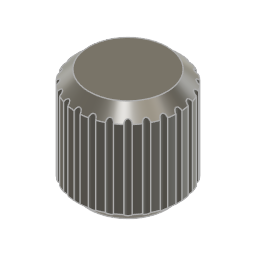
Shrimple20 Keypad Knob (Autodesk Fusion 360 design; units mm, degrees)
Autodesk Fusion 360 part; units mm, degrees
sketch "Sketch1" plane through (0, 0, 0) normal (0, 1, 0) x (1, 0, 0)
  circle A0 centre (0, 0) radius 8.5
  dimension "d1" = 17
  constraint coincident A0.centre origin
  measures "d1" diameter of A0
extrude "Extrude1" add sketch "Sketch1" along normal blind 17
ref_plane "WorkPlane1" through (0, 14, 0) normal (0, 1, 0) x (1, 0, 0)
sketch "Sketch2" plane through (0, 14, 0) normal (0, 1, 0) x (1, 0, 0)
  circle A0 centre (0, 0) radius 3.05
  line L0 (-0.5, 3.0087) -> (-0.5, -3.0087)
  line L1 (0.5, -3.0087) -> (0.5, 3.0087)
  line L2 (-0.5, 0) -> (0.5, 0) construction
  dimension "d5" = 6.1
  dimension "d6" = 1
  constraint coincident A0.centre origin
  constraint coincident A0 L0.start
  constraint coincident A0 L0.end
  constraint vertical L0
  constraint coincident A0 L1.start
  constraint coincident A0 L1.end
  constraint parallel L0 L1
  constraint midpoint L0 L2.start
  constraint midpoint L1 L2.end
  constraint midpoint A0.centre L2
  measures "d5" diameter of A0
  measures "d6" distance of L2.start L2.end
extrude "Extrude2" cut sketch "Sketch2" against normal blind 5 contours A0 L1 | A0 L0
sketch "Sketch3" plane through (0, 0, 0) normal (0, -1, 0) x (1, 0, 0)
  circle A0 centre (0, 0) radius 8.5
  circle A1 centre (0, 0) radius 4
  dimension "d9" = 8
  constraint coincident A0.centre A1.centre
  measures "d9" diameter of A1
extrude "Extrude3" cut sketch "Sketch3" against normal up to surface (9 mm away) contours A1
chamfer "Chamfer1" distance 0.95 angle 45 1 edges at (-3.7293, 9, 1.4465)
chamfer "Chamfer2" distance 2 angle 45 3 edges at (-3.7293, 0, 1.4465) (-7.9248, 0, 3.0737) (-7.9248, 17, 3.0737)
sketch "Sketch4" plane through (0, 17, 0) normal (0, 1, 0) x (-1, 0, 0)
  circle A0 centre (0, 0) radius 6.5
  circle A1 centre (0, 0) radius 8.5 construction
  line L0 (0, 0) -> (-8.5, 0) construction
  circle A2 centre (-8.5, 0) radius 0.5
  dimension "d14" = 1
  constraint coincident A0.centre A1.centre
  constraint coincident A1 L0.end
  constraint horizontal L0
  constraint coincident L0.end A2.centre
  measures "d14" diameter of A2
extrude "Extrude4" cut sketch "Sketch4" against normal blind 17 contours A2
pattern_circular "C-Pattern1" count 24 over 360 about axis through (0, 1.75, 0) along (0, 1, 0) of "Extrude4"
